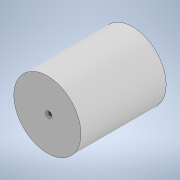
# Autodesk Inventor part: Media container
Saved by Autodesk Inventor 2021.3 (Build 253353010, 353A)
## iProperties
Created: 2021-07-06
Part Number: Media container
Material: Generic
Document SubType Name: Modeling
Designer: Dell
Density: 1 g/cm^3
Appearance: Default
Author: Dell
Autodesk Inventor part; units mm, degrees
ref_plane "YZ Plane" through (0, 0, 0) normal (1, 0, 0) x (0, 1, 0)
ref_plane "XZ Plane" through (0, 0, 0) normal (0, 1, 0) x (-1, 0, 0)
ref_plane "XY Plane" through (0, 0, 0) normal (0, 0, 1) x (1, 0, 0)
sketch "Sketch1" plane through (0, 0, 0) normal (0, 0, 1) x (1, 0, 0)
  circle A0 centre (0, 0) radius 50
  dimension "d0" = 100
  constraints: 1 centre point, 1 coincident
  measures "d0" diameter of A0
extrude "Extrusion1" add sketch "Sketch1" along normal blind 127
sketch "Sketch2" plane through (0, 0, 0) normal (0, 0, -1) x (-1, 0, 0)
  point P0 (0, 0)
  point P1 (3.0158, -0.2622)
hole "Hole1" at (-3.0158, -0.2622, 0) direction (0, 0, -1) diameter 5 depth 25.4 tip angle 118
sketch "Sketch3" plane through (0, 0, 127) normal (0, 0, 1) x (1, 0, 0)
  point P0 (0, 0)
  point P1 (2.1463, 0.878)
hole "Hole2" at (2.1463, 0.878, 127) direction (0, 0, -1) diameter 4.9784 depth 19.05 countersink diameter 9.525 countersink angle 82 thread size "1/4-20 UNC" class "2B" standard "ANSI Unified Screw Threads"
body "Solid1"
